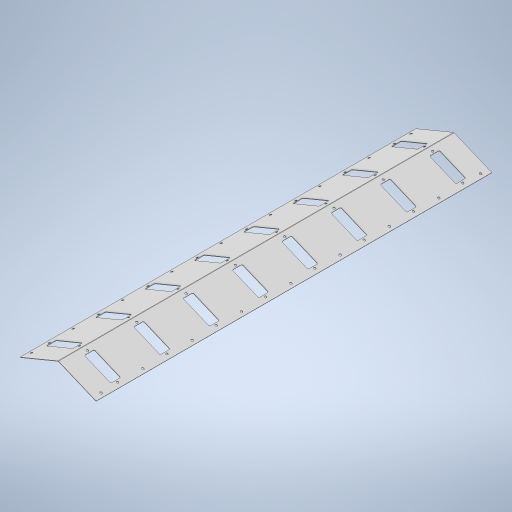
# Autodesk Inventor part: ДМФ 01 11 Барабан Лист крышка
Saved by Autodesk Inventor 2024.2 (Build 282272000, 272)
## iProperties
Created: 2024-04-28
Part Number: ДМФ 01 11 Барабан Лист крышка
Material: Generic
Document SubType Name: Sheet Metal
Designer: pokla
Density: 1 g/cm^3
Appearance: Default
Sheet Metal Rule: Default
Sheet Metal Width: 416,332 mm
Sheet Metal Length: 2006,000 mm
Sheet Metal Area: 835162,721 mm^2
Flat Pattern Width: 41.6332 cm
Flat Pattern Length: 200.6 cm
Flat Pattern Area: 8351.63 cm^2
Author: pokla
Autodesk Inventor part; units mm, degrees
ref_plane "YZ Plane" through (0, 0, 0) normal (1, 0, 0) x (0, 1, 0)
ref_plane "XZ Plane" through (0, 0, 0) normal (0, 1, 0) x (-1, 0, 0)
ref_plane "XY Plane" through (0, 0, 0) normal (0, 0, 1) x (1, 0, 0)
sketch "Sketch1" plane through (0, 0, 0) normal (0, 0, 1) x (1, 0, 0)
  line L0 (-193.637817, 193.637817) -> (0, 273.845227) construction
  line L1 (0, 273.845227) -> (193.637817, 193.637817) construction
  line L2 (193.637817, 193.637817) -> (273.845227, 0) construction
  line L3 (273.845227, 0) -> (193.637817, -193.637817) construction
  line L4 (193.637817, -193.637817) -> (0, -273.845227) construction
  line L5 (0, -273.845227) -> (-193.637817, -193.637817) construction
  line L6 (-193.637817, -193.637817) -> (-273.845227, 0) construction
  line L7 (-273.845227, 0) -> (-193.637817, 193.637817) construction
  line L8 (1.530734, 273.211176) -> (192.806325, 193.982232)
  line L9 (-1.530734, 273.211176) -> (-192.806325, 193.982232)
  arc A0 (1.530734, 273.211176) -> (-1.530734, 273.211176) centre (0, 269.515658) ccw
  point P0 (0, 0)
  point P1 (0, 0)
  dimension "d46" = 506
  dimension "d47" = 0.9
  dimension "d48" = 4
  measures "d46" distance between parallel lines of L7 L3
  measures "d47" distance of L0.start L9.end
  measures "d48" radius of A0
contour flange "Contour Flange2" sketch "Sketch1" thickness 2 bend radius 2 width 2006 along (0, 0, -1) mid plane no both sides no wall seen from (97.168529, 233.596704, 0) lies toward (-0.3826834, -0.9238795, 0) curves L8 A0 L9
bend "Bend4"
corner "Corner4"
sketch "Sketch12" plane through (1.530734, 273.211176, 0) normal (0.3826834, 0.9238795, 0) x (0.9238795, -0.3826834, 0)
  circle A0 centre (189.129, 40.75) radius 5.5
  line L0 (0, 0) -> (0, 2006)
  line L1 (207.035208, 0) -> (0, 0)
  circle A1 centre (189.129, 1965.25) radius 5.5
  line L2 (207.035208, 2006) -> (0, 2006)
  point P0 (103.139177, 0)
  dimension "d115" = 11
  dimension "d116" = 189.129
  dimension "d117" = 40.75
  dimension "d118" = 11
  dimension "d119" = 189.129
  dimension "d120" = 40.75
  constraints: 2 centre point
  measures "d115" diameter of A0
  measures "d116" distance from line of L0 A0.centre
  measures "d117" distance from line of L1 A0.centre
  measures "d118" diameter of A1
  measures "d119" distance from line of L0 A1.centre
  measures "d120" distance from line of L2 A1.centre
extrude "Extrusion5" cut sketch "Sketch12" against normal up to surface (2 mm away)
sketch "Sketch14" plane through (1.530734, 273.211176, 0) normal (0.3826834, 0.9238795, 0) x (0.9238795, -0.3826834, 0)
  line L0 (30.639, 1103) -> (175.639, 1103)
  line L1 (175.639, 1103) -> (175.639, 1153)
  line L2 (175.639, 1153) -> (30.639, 1153)
  line L3 (30.639, 1153) -> (30.639, 1103)
  circle A0 centre (20.639, 1128) radius 5
  circle A1 centre (185.639, 1128) radius 5
  line L4 (103.139, 1103) -> (103.139, 1153) construction
  line L5 (0, 0) -> (0, 2006) construction
  point P0 (103.139177, 0)
  point P1 (30.639, 1128)
  point P2 (175.639, 1128)
  point P3 (0, 1003)
  dimension "d131" = 145
  dimension "d132" = 50
  dimension "d133" = 10
  dimension "d134" = 10
  dimension "d135" = 125
  dimension "d136" = 103.139
  constraints: 10 end point, 5 midpoint, 2 centre point, 2 horizontal alignment, 2 parallel, 1 horizontal, 1 perpendicular, 1 other
  measures "d131" distance of L1.end L2.end
  measures "d132" distance of L2.end L0.start
  measures "d133" diameter of A0
  measures "d134" distance from line of L3 A0.centre
  measures "d135" vertical distance of point (0, 1003) point (30.639, 1128)
  measures "d136" distance from line of L5 L4.start
extrude "Extrusion7" cut sketch "Sketch14" against normal up to surface (2 mm away)
fillet "Fillet2" radius 5 4 edges at (29.4548, 260.5623, -1153) (29.4548, 260.5623, -1103) (163.4173, 205.0732, -1103) (163.4173, 205.0732, -1153)
pattern_circular "Circular Pattern1" count 2 over 45 about axis through (0, 0, -10) along (0, 0, 1) of "Extrusion7", "Fillet2"
pattern_linear "Rectangular Pattern5" count 8 spacing 250 along (0, 0, 1) of "Extrusion7", "Fillet2", "Circular Pattern1" first direction both ways yes
sketch "Sketch15" plane through (1.530734, 273.211176, 0) normal (0.3826834, 0.9238795, 0) x (0.9238795, -0.3826834, 0)
  circle A0 centre (189.129, 1003) radius 5.5
  line L0 (0, 0) -> (0, 2006) projected
  point P0 (103.139177, 0)
  point P1 (0, 1003)
  dimension "d146" = 11
  dimension "d147" = 189.129
  constraints: 1 centre point, 1 horizontal alignment, 1 midpoint
  measures "d146" diameter of A0
  measures "d147" distance from line of L0 A0.centre
extrude "Extrusion8" cut sketch "Sketch15" against normal through all
pattern_linear "Rectangular Pattern6" count 7 spacing 250 along (0, 0, 1) of "Extrusion8" first direction both ways yes
mirror "Mirror5" about plane through (0, 0, 0) normal (1, 0, 0) of "Extrusion8", "Extrusion5", "Rectangular Pattern6"
chamfer "Corner Chamfer1" distance 2 angle 45 1 edges at (-192.4236, 193.0584, 0)
fillet "Corner Round1" radius 2 1 edges at (192.4236, 193.0584, 0)
equation "\"d135\" = Отступ_окна_от_середины"
equation "\"d46\" = Барабан_габарит_по_кассетам"
equation "\"d47\" = Барабан_отступ_развертки"
equation "\"d48\" = BendRadius + Thickness"
equation "\"d118\" = d115"
equation "\"d119\" = d116"
equation "\"d120\" = d117"
equation "\"d131\" = Длина_окна_барабан"
equation "\"d132\" = Ширина_окна_барабан"
equation "\"d133\" = Диам_шпильки_под_кассету"
equation "\"d136\" = Расст_утановки_окна"
equation "\"d49\" = Thickness"
equation "\"d50\" = BendReliefWidth"
equation "\"d51\" = BendReliefDepth"
equation "\"d52\" = MinimumRemnant"
equation "\"d53\" = TransitionRadius"
equation "\"d54\" = Барабан_длина_листа"
equation "\"d55\" = BendRadius"
equation "\"d57\" = CornerReliefSize"
equation "\"d58\" = GapSize"
equation "\"d59\" = JacobiRadiusSize"
equation "\"BendRadius\" = Thickness"
equation "\"BendReliefWidth\" = Thickness"
equation "\"BendReliefDepth\" = 0.5 * Thickness"
equation "\"CornerReliefSize\" = 4 * Thickness"
equation "\"MinimumRemnant\" = 2 * Thickness"
equation "\"TransitionRadius\" = BendRadius"
equation "\"JacobiRadiusSize\" = BendRadius"
equation "\"GapSize\" = Thickness"
equation "\"Барабан_габарит_по_кассетам\" = 506"
equation "\"Барабан_отступ_развертки\" = 0.9"
equation "\"Thickness\" = 2"
equation "\"Длина_окна_барабан\" = 145"
equation "\"Ширина_окна_барабан\" = 50"
equation "\"Диам_шпильки_под_кассету\" = 10"
equation "\"Расст_утановки_окна\" = 103.139"
equation "\"Барабан_длина_листа\" = 2006"
equation "\"Отступ_окна_от_середины\" = 125"
body "Solid2"
